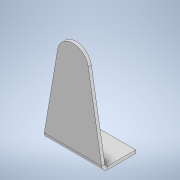
# Autodesk Inventor part: soporte_barra
Saved by Autodesk Inventor 2021 (Build 250183000, 183)
## iProperties
Created: 2021-04-16
Part Number: soporte_barra
Material: Genérico
Document SubType Name: Chapa
Designer: Leonardo Fabio Mercado Benítez
Density: 1 g/cm^3
Sheet Metal Rule: Por defecto_mm
Appearance: Valor por defecto
Author: Leonardo Fabio Mercado Benítez
Autodesk Inventor part; units mm, degrees
ref_plane "YZ Plane" through (0, 0, 0) normal (1, 0, 0) x (0, 1, 0)
ref_plane "XZ Plane" through (0, 0, 0) normal (0, 1, 0) x (-1, 0, 0)
ref_plane "XY Plane" through (0, 0, 0) normal (0, 0, 1) x (1, 0, 0)
sketch "Boceto1" plane through (0, 0, 0) normal (0, 1, 0) x (-1, 0, 0)
  line L0 (-17.5, 8.5) -> (17.5, 8.5)
  line L1 (17.5, 8.5) -> (17.5, -8.5)
  line L2 (17.5, -8.5) -> (-17.5, -8.5)
  line L3 (-17.5, -8.5) -> (-17.5, 8.5)
  line L4 (-17.5, 8.5) -> (17.5, -8.5) construction
  line L5 (17.5, 8.5) -> (-17.5, -8.5) construction
  point P0 (0, 0)
  dimension "d0" = 35
  dimension "d1" = 17
  measures "d0" distance of L1.end L2.end
  measures "d1" distance of L0.end L1.end
extrude "Placa1" add sketch "Boceto1" along normal blind 1.9
sketch "Boceto2" plane through (17.5, 3.8, 10.4) normal (0, 0, 1) x (1, 0, 0)
  line L0 (-35, 0) -> (0, 0)
  line L1 (0, 0) -> (0, 56.2)
  line L2 (0, 56.2) -> (-35, 56.2)
  line L3 (-35, 56.2) -> (-35, 0)
  constraints: 6 end point, 1 horizontal, 1 perpendicular, 1 vertical
edge flange "Pestaña1" height 60 angle 90 thickness 1.9 bend radius 1.9 thickness toward (0, 0, 1) relief straight relief width 1.9 relief depth 0.95 edges at (0, 1.9, 8.5) wall of the first edge with corners at (-17.5, 3.8, 10.4) (17.5, 3.8, 10.4) (17.5, 60, 10.4) (-17.5, 60, 10.4)
bend "Doblez1"
corner "Esquina1"
sketch "Boceto3" plane through (-17.5, 60, 12.3) normal (0, 0, 1) x (1, 0, 0)
  arc A0 (26.8043, -7.9448) -> (8.1957, -7.9448) centre (17.5, -9.525) ccw
  line L0 (0, -56.2) -> (8.1957, -7.9448)
  line L1 (35, -56.2) -> (26.8043, -7.9448)
  line L2 (0, 0) -> (0, -56.2) projected
  line L3 (0, -56.2) -> (0, 0)
  line L4 (0, 0) -> (35, 0) projected
  line L5 (0, 0) -> (35, 0)
  line L6 (35, 0) -> (35, -56.2) projected
  line L7 (35, 0) -> (35, -56.2)
  point P0 (17.5, -60)
  dimension "d13" = 18.875
  constraints: 10 end point, 2 perpendicular, 2 point on circle, 2 tangent, 1 centre point, 1 vertical
  measures "d13" diameter of A0
extrude "Cortar1" cut sketch "Boceto3" against normal blind 1.9
equation "\"d16\" = Grosor"
equation "\"d2\" = Grosor"
equation "\"d3\" = Anchura_desahogo_plegado"
equation "\"d4\" = Profundidad_desahogo_plegado"
equation "\"d5\" = Remanente_mínimo"
equation "\"d6\" = Radiodetransición"
equation "\"d9\" = Radio_pliegue"
equation "\"d10\" = Tamaño_destalonado"
equation "\"d11\" = TamañoSeparación"
equation "\"d12\" = Tamaño_de_radio_de_Jacobi"
equation "\"Radio_pliegue\" = Grosor"
equation "\"Anchura_desahogo_plegado\" = Grosor"
equation "\"Profundidad_desahogo_plegado\" = 0.5 * Grosor"
equation "\"Tamaño_destalonado\" = 4 * Grosor"
equation "\"Remanente_mínimo\" = 2 * Grosor"
equation "\"Radiodetransición\" = Radio_pliegue"
equation "\"Tamaño_de_radio_de_Jacobi\" = Radio_pliegue"
equation "\"TamañoSeparación\" = Grosor"
equation "\"Grosor\" = 1.9"
